Autodesk Inventor part; units mm, degrees
(part 2 of 3)
  line L756 (23.8125, 171.1325) -> (24.4475, 171.1325)
  line L757 (24.4475, 171.1325) -> (24.4475, 171.7675)
  line L758 (23.8125, 171.7675) -> (23.8125, 171.1325)
  line L759 (24.4475, 171.7675) -> (23.8125, 171.7675)
  line L760 (24.4475, 171.7675) -> (23.8125, 171.1325) construction
  line L761 (23.8125, 171.7675) -> (24.4475, 171.1325) construction
  line L762 (26.3525, 171.1325) -> (26.9875, 171.1325)
  line L763 (26.9875, 171.1325) -> (26.9875, 171.7675)
  line L764 (26.3525, 171.7675) -> (26.3525, 171.1325)
  line L765 (26.9875, 171.7675) -> (26.3525, 171.7675)
  line L766 (26.9875, 171.7675) -> (26.3525, 171.1325) construction
  line L767 (26.3525, 171.7675) -> (26.9875, 171.1325) construction
  line L768 (28.8925, 171.1325) -> (29.5275, 171.1325)
  line L769 (29.5275, 171.1325) -> (29.5275, 171.7675)
  line L770 (28.8925, 171.7675) -> (28.8925, 171.1325)
  line L771 (29.5275, 171.7675) -> (28.8925, 171.7675)
  line L772 (29.5275, 171.7675) -> (28.8925, 171.1325) construction
  line L773 (28.8925, 171.7675) -> (29.5275, 171.1325) construction
  line L774 (31.4325, 171.1325) -> (32.0675, 171.1325)
  line L775 (32.0675, 171.1325) -> (32.0675, 171.7675)
  line L776 (31.4325, 171.7675) -> (31.4325, 171.1325)
  line L777 (32.0675, 171.7675) -> (31.4325, 171.7675)
  line L778 (32.0675, 171.7675) -> (31.4325, 171.1325) construction
  line L779 (31.4325, 171.7675) -> (32.0675, 171.1325) construction
  line L780 (33.9725, 171.1325) -> (34.6075, 171.1325)
  line L781 (34.6075, 171.1325) -> (34.6075, 171.7675)
  line L782 (33.9725, 171.7675) -> (33.9725, 171.1325)
  line L783 (34.6075, 171.7675) -> (33.9725, 171.7675)
  line L784 (34.6075, 171.7675) -> (33.9725, 171.1325) construction
  line L785 (33.9725, 171.7675) -> (34.6075, 171.1325) construction
  line L786 (36.5125, 171.1325) -> (37.1475, 171.1325)
  line L787 (37.1475, 171.1325) -> (37.1475, 171.7675)
  line L788 (36.5125, 171.7675) -> (36.5125, 171.1325)
  line L789 (37.1475, 171.7675) -> (36.5125, 171.7675)
  line L790 (37.1475, 171.7675) -> (36.5125, 171.1325) construction
  line L791 (36.5125, 171.7675) -> (37.1475, 171.1325) construction
  line L792 (39.0525, 171.1325) -> (39.6875, 171.1325)
  line L793 (39.6875, 171.1325) -> (39.6875, 171.7675)
  line L794 (39.0525, 171.7675) -> (39.0525, 171.1325)
  line L795 (39.6875, 171.7675) -> (39.0525, 171.7675)
  line L796 (39.6875, 171.7675) -> (39.0525, 171.1325) construction
  line L797 (39.0525, 171.7675) -> (39.6875, 171.1325) construction
  line L798 (169.2275, 37.1475) -> (168.5925, 37.1475)
  line L799 (168.5925, 36.5125) -> (169.2275, 36.5125)
  line L800 (169.2275, 36.5125) -> (169.2275, 37.1475)
  line L801 (169.2275, 37.1475) -> (168.5925, 36.5125) construction
  line L802 (168.5925, 37.1475) -> (169.2275, 36.5125) construction
  line L803 (168.5925, 37.1475) -> (168.5925, 36.5125)
  line L804 (169.2275, 34.6075) -> (168.5925, 34.6075)
  line L805 (168.5925, 33.9725) -> (169.2275, 33.9725)
  line L806 (169.2275, 33.9725) -> (169.2275, 34.6075)
  line L807 (169.2275, 34.6075) -> (168.5925, 33.9725) construction
  line L808 (168.5925, 34.6075) -> (169.2275, 33.9725) construction
  line L809 (168.5925, 34.6075) -> (168.5925, 33.9725)
  line L810 (169.2275, 32.0675) -> (168.5925, 32.0675)
  line L811 (168.5925, 31.4325) -> (169.2275, 31.4325)
  line L812 (169.2275, 31.4325) -> (169.2275, 32.0675)
  line L813 (169.2275, 32.0675) -> (168.5925, 31.4325) construction
  line L814 (168.5925, 32.0675) -> (169.2275, 31.4325) construction
  line L815 (168.5925, 32.0675) -> (168.5925, 31.4325)
  line L816 (169.2275, 29.5275) -> (168.5925, 29.5275)
  line L817 (168.5925, 28.8925) -> (169.2275, 28.8925)
  line L818 (169.2275, 28.8925) -> (169.2275, 29.5275)
  line L819 (169.2275, 29.5275) -> (168.5925, 28.8925) construction
  line L820 (168.5925, 29.5275) -> (169.2275, 28.8925) construction
  line L821 (168.5925, 29.5275) -> (168.5925, 28.8925)
  line L822 (169.2275, 26.9875) -> (168.5925, 26.9875)
  line L823 (168.5925, 26.3525) -> (169.2275, 26.3525)
  line L824 (169.2275, 26.3525) -> (169.2275, 26.9875)
  line L825 (169.2275, 26.9875) -> (168.5925, 26.3525) construction
  line L826 (168.5925, 26.9875) -> (169.2275, 26.3525) construction
  line L827 (168.5925, 26.9875) -> (168.5925, 26.3525)
  line L828 (169.2275, 24.4475) -> (168.5925, 24.4475)
  line L829 (168.5925, 23.8125) -> (169.2275, 23.8125)
  line L830 (169.2275, 23.8125) -> (169.2275, 24.4475)
  line L831 (169.2275, 24.4475) -> (168.5925, 23.8125) construction
  line L832 (168.5925, 24.4475) -> (169.2275, 23.8125) construction
  line L833 (168.5925, 24.4475) -> (168.5925, 23.8125)
  line L834 (169.2275, 21.9075) -> (168.5925, 21.9075)
  line L835 (168.5925, 21.2725) -> (169.2275, 21.2725)
  line L836 (169.2275, 21.2725) -> (169.2275, 21.9075)
  line L837 (169.2275, 21.9075) -> (168.5925, 21.2725) construction
  line L838 (168.5925, 21.9075) -> (169.2275, 21.2725) construction
  line L839 (168.5925, 21.9075) -> (168.5925, 21.2725)
  line L840 (169.2275, 19.3675) -> (168.5925, 19.3675)
  line L841 (168.5925, 18.7325) -> (169.2275, 18.7325)
  line L842 (169.2275, 18.7325) -> (169.2275, 19.3675)
  line L843 (169.2275, 19.3675) -> (168.5925, 18.7325) construction
  line L844 (168.5925, 19.3675) -> (169.2275, 18.7325) construction
  line L845 (168.5925, 19.3675) -> (168.5925, 18.7325)
  line L846 (169.2275, 16.8275) -> (168.5925, 16.8275)
  line L847 (168.5925, 16.1925) -> (169.2275, 16.1925)
  line L848 (169.2275, 16.1925) -> (169.2275, 16.8275)
  line L849 (169.2275, 16.8275) -> (168.5925, 16.1925) construction
  line L850 (168.5925, 16.8275) -> (169.2275, 16.1925) construction
  line L851 (168.5925, 16.8275) -> (168.5925, 16.1925)
  line L852 (169.2275, 14.2875) -> (168.5925, 14.2875)
  line L853 (168.5925, 13.6525) -> (169.2275, 13.6525)
  line L854 (169.2275, 13.6525) -> (169.2275, 14.2875)
  line L855 (169.2275, 14.2875) -> (168.5925, 13.6525) construction
  line L856 (168.5925, 14.2875) -> (169.2275, 13.6525) construction
  line L857 (168.5925, 14.2875) -> (168.5925, 13.6525)
  line L858 (169.2275, 11.7475) -> (168.5925, 11.7475)
  line L859 (168.5925, 11.1125) -> (169.2275, 11.1125)
  line L860 (169.2275, 11.1125) -> (169.2275, 11.7475)
  line L861 (169.2275, 11.7475) -> (168.5925, 11.1125) construction
  line L862 (168.5925, 11.7475) -> (169.2275, 11.1125) construction
  line L863 (168.5925, 11.7475) -> (168.5925, 11.1125)
  line L864 (169.2275, 9.2075) -> (168.5925, 9.2075)
  line L865 (168.5925, 8.5725) -> (169.2275, 8.5725)
  line L866 (169.2275, 8.5725) -> (169.2275, 9.2075)
  line L867 (169.2275, 9.2075) -> (168.5925, 8.5725) construction
  line L868 (168.5925, 9.2075) -> (169.2275, 8.5725) construction
  line L869 (168.5925, 9.2075) -> (168.5925, 8.5725)
  line L870 (169.2275, 6.6675) -> (168.5925, 6.6675)
  line L871 (168.5925, 6.0325) -> (169.2275, 6.0325)
  line L872 (169.2275, 6.0325) -> (169.2275, 6.6675)
  line L873 (169.2275, 6.6675) -> (168.5925, 6.0325) construction
  line L874 (168.5925, 6.6675) -> (169.2275, 6.0325) construction
  line L875 (168.5925, 6.6675) -> (168.5925, 6.0325)
  line L876 (169.2275, 4.1275) -> (168.5925, 4.1275)
  line L877 (168.5925, 3.4925) -> (169.2275, 3.4925)
  line L878 (169.2275, 3.4925) -> (169.2275, 4.1275)
  line L879 (169.2275, 4.1275) -> (168.5925, 3.4925) construction
  line L880 (168.5925, 4.1275) -> (169.2275, 3.4925) construction
  line L881 (168.5925, 4.1275) -> (168.5925, 3.4925)
  line L882 (169.2275, 1.5875) -> (168.5925, 1.5875)
  line L883 (168.5925, 0.9525) -> (169.2275, 0.9525)
  line L884 (169.2275, 0.9525) -> (169.2275, 1.5875)
  line L885 (169.2275, 1.5875) -> (168.5925, 0.9525) construction
  line L886 (168.5925, 1.5875) -> (169.2275, 0.9525) construction
  line L887 (168.5925, 1.5875) -> (168.5925, 0.9525)
  line L888 (169.2275, -0.9525) -> (168.5925, -0.9525)
  line L889 (168.5925, -1.5875) -> (169.2275, -1.5875)
  line L890 (169.2275, -1.5875) -> (169.2275, -0.9525)
  line L891 (169.2275, -0.9525) -> (168.5925, -1.5875) construction
  line L892 (168.5925, -0.9525) -> (169.2275, -1.5875) construction
  line L893 (168.5925, -0.9525) -> (168.5925, -1.5875)
  line L894 (169.2275, -3.4925) -> (168.5925, -3.4925)
  line L895 (168.5925, -4.1275) -> (169.2275, -4.1275)
  line L896 (169.2275, -4.1275) -> (169.2275, -3.4925)
  line L897 (169.2275, -3.4925) -> (168.5925, -4.1275) construction
  line L898 (168.5925, -3.4925) -> (169.2275, -4.1275) construction
  line L899 (168.5925, -3.4925) -> (168.5925, -4.1275)
  line L900 (169.2275, -6.0325) -> (168.5925, -6.0325)
  line L901 (168.5925, -6.6675) -> (169.2275, -6.6675)
  line L902 (169.2275, -6.6675) -> (169.2275, -6.0325)
  line L903 (169.2275, -6.0325) -> (168.5925, -6.6675) construction
  line L904 (168.5925, -6.0325) -> (169.2275, -6.6675) construction
  line L905 (168.5925, -6.0325) -> (168.5925, -6.6675)
  line L906 (169.2275, -8.5725) -> (168.5925, -8.5725)
  line L907 (168.5925, -9.2075) -> (169.2275, -9.2075)
  line L908 (169.2275, -9.2075) -> (169.2275, -8.5725)
  line L909 (169.2275, -8.5725) -> (168.5925, -9.2075) construction
  line L910 (168.5925, -8.5725) -> (169.2275, -9.2075) construction
  line L911 (168.5925, -8.5725) -> (168.5925, -9.2075)
  line L912 (169.2275, -11.1125) -> (168.5925, -11.1125)
  line L913 (168.5925, -11.7475) -> (169.2275, -11.7475)
  line L914 (169.2275, -11.7475) -> (169.2275, -11.1125)
  line L915 (169.2275, -11.1125) -> (168.5925, -11.7475) construction
  line L916 (168.5925, -11.1125) -> (169.2275, -11.7475) construction
  line L917 (168.5925, -11.1125) -> (168.5925, -11.7475)
  line L918 (169.2275, -13.6525) -> (168.5925, -13.6525)
  line L919 (168.5925, -14.2875) -> (169.2275, -14.2875)
  line L920 (169.2275, -14.2875) -> (169.2275, -13.6525)
  line L921 (169.2275, -13.6525) -> (168.5925, -14.2875) construction
  line L922 (168.5925, -13.6525) -> (169.2275, -14.2875) construction
  line L923 (168.5925, -13.6525) -> (168.5925, -14.2875)
  line L924 (169.2275, -16.1925) -> (168.5925, -16.1925)
  line L925 (168.5925, -16.8275) -> (169.2275, -16.8275)
  line L926 (169.2275, -16.8275) -> (169.2275, -16.1925)
  line L927 (169.2275, -16.1925) -> (168.5925, -16.8275) construction
  line L928 (168.5925, -16.1925) -> (169.2275, -16.8275) construction
  line L929 (168.5925, -16.1925) -> (168.5925, -16.8275)
  line L930 (169.2275, -18.7325) -> (168.5925, -18.7325)
  line L931 (168.5925, -19.3675) -> (169.2275, -19.3675)
  line L932 (169.2275, -19.3675) -> (169.2275, -18.7325)
  line L933 (169.2275, -18.7325) -> (168.5925, -19.3675) construction
  line L934 (168.5925, -18.7325) -> (169.2275, -19.3675) construction
  line L935 (168.5925, -18.7325) -> (168.5925, -19.3675)
  line L936 (169.2275, -21.2725) -> (168.5925, -21.2725)
  line L937 (168.5925, -21.9075) -> (169.2275, -21.9075)
  line L938 (169.2275, -21.9075) -> (169.2275, -21.2725)
  line L939 (169.2275, -21.2725) -> (168.5925, -21.9075) construction
  line L940 (168.5925, -21.2725) -> (169.2275, -21.9075) construction
  line L941 (168.5925, -21.2725) -> (168.5925, -21.9075)
  line L942 (169.2275, -23.8125) -> (168.5925, -23.8125)
  line L943 (168.5925, -24.4475) -> (169.2275, -24.4475)
  line L944 (169.2275, -24.4475) -> (169.2275, -23.8125)
  line L945 (169.2275, -23.8125) -> (168.5925, -24.4475) construction
  line L946 (168.5925, -23.8125) -> (169.2275, -24.4475) construction
  line L947 (168.5925, -23.8125) -> (168.5925, -24.4475)
  line L948 (169.2275, -26.3525) -> (168.5925, -26.3525)
  line L949 (168.5925, -26.9875) -> (169.2275, -26.9875)
  line L950 (169.2275, -26.9875) -> (169.2275, -26.3525)
  line L951 (169.2275, -26.3525) -> (168.5925, -26.9875) construction
  line L952 (168.5925, -26.3525) -> (169.2275, -26.9875) construction
  line L953 (168.5925, -26.3525) -> (168.5925, -26.9875)
  line L954 (169.2275, -28.8925) -> (168.5925, -28.8925)
  line L955 (168.5925, -29.5275) -> (169.2275, -29.5275)
  line L956 (169.2275, -29.5275) -> (169.2275, -28.8925)
  line L957 (169.2275, -28.8925) -> (168.5925, -29.5275) construction
  line L958 (168.5925, -28.8925) -> (169.2275, -29.5275) construction
  line L959 (168.5925, -28.8925) -> (168.5925, -29.5275)
  line L960 (169.2275, -31.4325) -> (168.5925, -31.4325)
  line L961 (168.5925, -32.0675) -> (169.2275, -32.0675)
  line L962 (169.2275, -32.0675) -> (169.2275, -31.4325)
  line L963 (169.2275, -31.4325) -> (168.5925, -32.0675) construction
  line L964 (168.5925, -31.4325) -> (169.2275, -32.0675) construction
  line L965 (168.5925, -31.4325) -> (168.5925, -32.0675)
  line L966 (169.2275, -33.9725) -> (168.5925, -33.9725)
  line L967 (168.5925, -34.6075) -> (169.2275, -34.6075)
  line L968 (169.2275, -34.6075) -> (169.2275, -33.9725)
  line L969 (169.2275, -33.9725) -> (168.5925, -34.6075) construction
  line L970 (168.5925, -33.9725) -> (169.2275, -34.6075) construction
  line L971 (168.5925, -33.9725) -> (168.5925, -34.6075)
  line L972 (169.2275, -36.5125) -> (168.5925, -36.5125)
  line L973 (168.5925, -37.1475) -> (169.2275, -37.1475)
  line L974 (169.2275, -37.1475) -> (169.2275, -36.5125)
  line L975 (169.2275, -36.5125) -> (168.5925, -37.1475) construction
  line L976 (168.5925, -36.5125) -> (169.2275, -37.1475) construction
  line L977 (168.5925, -36.5125) -> (168.5925, -37.1475)
  line L978 (169.2275, -39.0525) -> (168.5925, -39.0525)
  line L979 (168.5925, -39.6875) -> (169.2275, -39.6875)
  line L980 (169.2275, -39.6875) -> (169.2275, -39.0525)
  line L981 (169.2275, -39.0525) -> (168.5925, -39.6875) construction
  line L982 (168.5925, -39.0525) -> (169.2275, -39.6875) construction
  line L983 (168.5925, -39.0525) -> (168.5925, -39.6875)
  line L984 (171.7675, 39.6875) -> (171.1325, 39.6875)
  line L985 (171.1325, 39.0525) -> (171.7675, 39.0525)
  line L986 (171.7675, 39.0525) -> (171.7675, 39.6875)
  line L987 (171.7675, 39.6875) -> (171.1325, 39.0525) construction
  line L988 (171.1325, 39.6875) -> (171.7675, 39.0525) construction
  line L989 (171.1325, 39.6875) -> (171.1325, 39.0525)
  line L990 (171.7675, 37.1475) -> (171.1325, 37.1475)
  line L991 (171.1325, 36.5125) -> (171.7675, 36.5125)
  line L992 (171.7675, 36.5125) -> (171.7675, 37.1475)
  line L993 (171.7675, 37.1475) -> (171.1325, 36.5125) construction
  line L994 (171.1325, 37.1475) -> (171.7675, 36.5125) construction
  line L995 (171.1325, 37.1475) -> (171.1325, 36.5125)
  line L996 (171.7675, 34.6075) -> (171.1325, 34.6075)
  line L997 (171.1325, 33.9725) -> (171.7675, 33.9725)
  line L998 (171.7675, 33.9725) -> (171.7675, 34.6075)
  line L999 (171.7675, 34.6075) -> (171.1325, 33.9725) construction
  line L1000 (171.1325, 34.6075) -> (171.7675, 33.9725) construction
  line L1001 (171.1325, 34.6075) -> (171.1325, 33.9725)
  line L1002 (171.7675, 32.0675) -> (171.1325, 32.0675)
  line L1003 (171.1325, 31.4325) -> (171.7675, 31.4325)
  line L1004 (171.7675, 31.4325) -> (171.7675, 32.0675)
  line L1005 (171.7675, 32.0675) -> (171.1325, 31.4325) construction
  line L1006 (171.1325, 32.0675) -> (171.7675, 31.4325) construction
  line L1007 (171.1325, 32.0675) -> (171.1325, 31.4325)
  line L1008 (171.7675, 29.5275) -> (171.1325, 29.5275)
  line L1009 (171.1325, 28.8925) -> (171.7675, 28.8925)
  line L1010 (171.7675, 28.8925) -> (171.7675, 29.5275)
  line L1011 (171.7675, 29.5275) -> (171.1325, 28.8925) construction
  line L1012 (171.1325, 29.5275) -> (171.7675, 28.8925) construction
  line L1013 (171.1325, 29.5275) -> (171.1325, 28.8925)
  line L1014 (171.7675, 26.9875) -> (171.1325, 26.9875)
  line L1015 (171.1325, 26.3525) -> (171.7675, 26.3525)
  line L1016 (171.7675, 26.3525) -> (171.7675, 26.9875)
  line L1017 (171.7675, 26.9875) -> (171.1325, 26.3525) construction
  line L1018 (171.1325, 26.9875) -> (171.7675, 26.3525) construction
  line L1019 (171.1325, 26.9875) -> (171.1325, 26.3525)
  line L1020 (171.7675, 24.4475) -> (171.1325, 24.4475)
  line L1021 (171.1325, 23.8125) -> (171.7675, 23.8125)
  line L1022 (171.7675, 23.8125) -> (171.7675, 24.4475)
  line L1023 (171.7675, 24.4475) -> (171.1325, 23.8125) construction
  line L1024 (171.1325, 24.4475) -> (171.7675, 23.8125) construction
  line L1025 (171.1325, 24.4475) -> (171.1325, 23.8125)
  line L1026 (171.7675, 21.9075) -> (171.1325, 21.9075)
  line L1027 (171.1325, 21.2725) -> (171.7675, 21.2725)
  line L1028 (171.7675, 21.2725) -> (171.7675, 21.9075)
  line L1029 (171.7675, 21.9075) -> (171.1325, 21.2725) construction
  line L1030 (171.1325, 21.9075) -> (171.7675, 21.2725) construction
  line L1031 (171.1325, 21.9075) -> (171.1325, 21.2725)
  line L1032 (171.7675, 19.3675) -> (171.1325, 19.3675)
  line L1033 (171.1325, 18.7325) -> (171.7675, 18.7325)
  line L1034 (171.7675, 18.7325) -> (171.7675, 19.3675)
  line L1035 (171.7675, 19.3675) -> (171.1325, 18.7325) construction
  line L1036 (171.1325, 19.3675) -> (171.7675, 18.7325) construction
  line L1037 (171.1325, 19.3675) -> (171.1325, 18.7325)
  line L1038 (171.7675, 16.8275) -> (171.1325, 16.8275)
  line L1039 (171.1325, 16.1925) -> (171.7675, 16.1925)
  line L1040 (171.7675, 16.1925) -> (171.7675, 16.8275)
  line L1041 (171.7675, 16.8275) -> (171.1325, 16.1925) construction
  line L1042 (171.1325, 16.8275) -> (171.7675, 16.1925) construction
  line L1043 (171.1325, 16.8275) -> (171.1325, 16.1925)
  line L1044 (171.7675, 14.2875) -> (171.1325, 14.2875)
  line L1045 (171.1325, 13.6525) -> (171.7675, 13.6525)
  line L1046 (171.7675, 13.6525) -> (171.7675, 14.2875)
  line L1047 (171.7675, 14.2875) -> (171.1325, 13.6525) construction
  line L1048 (171.1325, 14.2875) -> (171.7675, 13.6525) construction
  line L1049 (171.1325, 14.2875) -> (171.1325, 13.6525)
  line L1050 (171.7675, 11.7475) -> (171.1325, 11.7475)
  line L1051 (171.1325, 11.1125) -> (171.7675, 11.1125)
  line L1052 (171.7675, 11.1125) -> (171.7675, 11.7475)
  line L1053 (171.7675, 11.7475) -> (171.1325, 11.1125) construction
  line L1054 (171.1325, 11.7475) -> (171.7675, 11.1125) construction
  line L1055 (171.1325, 11.7475) -> (171.1325, 11.1125)
  line L1056 (171.7675, 9.2075) -> (171.1325, 9.2075)
  line L1057 (171.1325, 8.5725) -> (171.7675, 8.5725)
  line L1058 (171.7675, 8.5725) -> (171.7675, 9.2075)
  line L1059 (171.7675, 9.2075) -> (171.1325, 8.5725) construction
  line L1060 (171.1325, 9.2075) -> (171.7675, 8.5725) construction
  line L1061 (171.1325, 9.2075) -> (171.1325, 8.5725)
  line L1062 (171.7675, 6.6675) -> (171.1325, 6.6675)
  line L1063 (171.1325, 6.0325) -> (171.7675, 6.0325)
  line L1064 (171.7675, 6.0325) -> (171.7675, 6.6675)
  line L1065 (171.7675, 6.6675) -> (171.1325, 6.0325) construction
  line L1066 (171.1325, 6.6675) -> (171.7675, 6.0325) construction
  line L1067 (171.1325, 6.6675) -> (171.1325, 6.0325)
  line L1068 (171.7675, 4.1275) -> (171.1325, 4.1275)
  line L1069 (171.1325, 3.4925) -> (171.7675, 3.4925)
  line L1070 (171.7675, 3.4925) -> (171.7675, 4.1275)
  line L1071 (171.7675, 4.1275) -> (171.1325, 3.4925) construction
  line L1072 (171.1325, 4.1275) -> (171.7675, 3.4925) construction
  line L1073 (171.1325, 4.1275) -> (171.1325, 3.4925)
  line L1074 (171.7675, 1.5875) -> (171.1325, 1.5875)
  line L1075 (171.1325, 0.9525) -> (171.7675, 0.9525)
  line L1076 (171.7675, 0.9525) -> (171.7675, 1.5875)
  line L1077 (171.7675, 1.5875) -> (171.1325, 0.9525) construction
  line L1078 (171.1325, 1.5875) -> (171.7675, 0.9525) construction
  line L1079 (171.1325, 1.5875) -> (171.1325, 0.9525)
  line L1080 (171.7675, -0.9525) -> (171.1325, -0.9525)
  line L1081 (171.1325, -1.5875) -> (171.7675, -1.5875)
  line L1082 (171.7675, -1.5875) -> (171.7675, -0.9525)
  line L1083 (171.7675, -0.9525) -> (171.1325, -1.5875) construction
  line L1084 (171.1325, -0.9525) -> (171.7675, -1.5875) construction
  line L1085 (171.1325, -0.9525) -> (171.1325, -1.5875)
  line L1086 (171.7675, -3.4925) -> (171.1325, -3.4925)
  line L1087 (171.1325, -4.1275) -> (171.7675, -4.1275)
  line L1088 (171.7675, -4.1275) -> (171.7675, -3.4925)
  line L1089 (171.7675, -3.4925) -> (171.1325, -4.1275) construction
  line L1090 (171.1325, -3.4925) -> (171.7675, -4.1275) construction
  line L1091 (171.1325, -3.4925) -> (171.1325, -4.1275)
  line L1092 (171.7675, -6.0325) -> (171.1325, -6.0325)
  line L1093 (171.1325, -6.6675) -> (171.7675, -6.6675)
  line L1094 (171.7675, -6.6675) -> (171.7675, -6.0325)
  line L1095 (171.7675, -6.0325) -> (171.1325, -6.6675) construction
  line L1096 (171.1325, -6.0325) -> (171.7675, -6.6675) construction
  line L1097 (171.1325, -6.0325) -> (171.1325, -6.6675)
  line L1098 (171.7675, -8.5725) -> (171.1325, -8.5725)
  line L1099 (171.1325, -9.2075) -> (171.7675, -9.2075)
  line L1100 (171.7675, -9.2075) -> (171.7675, -8.5725)
  line L1101 (171.7675, -8.5725) -> (171.1325, -9.2075) construction
  line L1102 (171.1325, -8.5725) -> (171.7675, -9.2075) construction
  line L1103 (171.1325, -8.5725) -> (171.1325, -9.2075)
  line L1104 (171.7675, -11.1125) -> (171.1325, -11.1125)
  line L1105 (171.1325, -11.7475) -> (171.7675, -11.7475)
  line L1106 (171.7675, -11.7475) -> (171.7675, -11.1125)
  line L1107 (171.7675, -11.1125) -> (171.1325, -11.7475) construction
  line L1108 (171.1325, -11.1125) -> (171.7675, -11.7475) construction
  line L1109 (171.1325, -11.1125) -> (171.1325, -11.7475)
  line L1110 (171.7675, -13.6525) -> (171.1325, -13.6525)
  line L1111 (171.1325, -14.2875) -> (171.7675, -14.2875)
  line L1112 (171.7675, -14.2875) -> (171.7675, -13.6525)
  line L1113 (171.7675, -13.6525) -> (171.1325, -14.2875) construction
  line L1114 (171.1325, -13.6525) -> (171.7675, -14.2875) construction
  line L1115 (171.1325, -13.6525) -> (171.1325, -14.2875)
  line L1116 (171.7675, -16.1925) -> (171.1325, -16.1925)
  line L1117 (171.1325, -16.8275) -> (171.7675, -16.8275)
  line L1118 (171.7675, -16.8275) -> (171.7675, -16.1925)
  line L1119 (171.7675, -16.1925) -> (171.1325, -16.8275) construction
  line L1120 (171.1325, -16.1925) -> (171.7675, -16.8275) construction
  line L1121 (171.1325, -16.1925) -> (171.1325, -16.8275)
  line L1122 (171.7675, -18.7325) -> (171.1325, -18.7325)
  line L1123 (171.1325, -19.3675) -> (171.7675, -19.3675)
  line L1124 (171.7675, -19.3675) -> (171.7675, -18.7325)
  line L1125 (171.7675, -18.7325) -> (171.1325, -19.3675) construction
  line L1126 (171.1325, -18.7325) -> (171.7675, -19.3675) construction
  line L1127 (171.1325, -18.7325) -> (171.1325, -19.3675)
  line L1128 (171.7675, -21.2725) -> (171.1325, -21.2725)
  line L1129 (171.1325, -21.9075) -> (171.7675, -21.9075)
  line L1130 (171.7675, -21.9075) -> (171.7675, -21.2725)
  line L1131 (171.7675, -21.2725) -> (171.1325, -21.9075) construction
  line L1132 (171.1325, -21.2725) -> (171.7675, -21.9075) construction
  line L1133 (171.1325, -21.2725) -> (171.1325, -21.9075)
  line L1134 (171.7675, -23.8125) -> (171.1325, -23.8125)
  line L1135 (171.1325, -24.4475) -> (171.7675, -24.4475)
  line L1136 (171.7675, -24.4475) -> (171.7675, -23.8125)
  line L1137 (171.7675, -23.8125) -> (171.1325, -24.4475) construction
  line L1138 (171.1325, -23.8125) -> (171.7675, -24.4475) construction
  line L1139 (171.1325, -23.8125) -> (171.1325, -24.4475)
  line L1140 (171.7675, -26.3525) -> (171.1325, -26.3525)
  line L1141 (171.1325, -26.9875) -> (171.7675, -26.9875)
  line L1142 (171.7675, -26.9875) -> (171.7675, -26.3525)
  line L1143 (171.7675, -26.3525) -> (171.1325, -26.9875) construction
  line L1144 (171.1325, -26.3525) -> (171.7675, -26.9875) construction
  line L1145 (171.1325, -26.3525) -> (171.1325, -26.9875)
  line L1146 (171.7675, -28.8925) -> (171.1325, -28.8925)
  line L1147 (171.1325, -29.5275) -> (171.7675, -29.5275)
  line L1148 (171.7675, -29.5275) -> (171.7675, -28.8925)
  line L1149 (171.7675, -28.8925) -> (171.1325, -29.5275) construction
  line L1150 (171.1325, -28.8925) -> (171.7675, -29.5275) construction
  line L1151 (171.1325, -28.8925) -> (171.1325, -29.5275)
  line L1152 (171.7675, -31.4325) -> (171.1325, -31.4325)
  line L1153 (171.1325, -32.0675) -> (171.7675, -32.0675)
  line L1154 (171.7675, -32.0675) -> (171.7675, -31.4325)
  line L1155 (171.7675, -31.4325) -> (171.1325, -32.0675) construction
  line L1156 (171.1325, -31.4325) -> (171.7675, -32.0675) construction
  line L1157 (171.1325, -31.4325) -> (171.1325, -32.0675)
  line L1158 (171.7675, -33.9725) -> (171.1325, -33.9725)
  line L1159 (171.1325, -34.6075) -> (171.7675, -34.6075)
  line L1160 (171.7675, -34.6075) -> (171.7675, -33.9725)
  line L1161 (171.7675, -33.9725) -> (171.1325, -34.6075) construction
  line L1162 (171.1325, -33.9725) -> (171.7675, -34.6075) construction
  line L1163 (171.1325, -33.9725) -> (171.1325, -34.6075)
  line L1164 (171.7675, -36.5125) -> (171.1325, -36.5125)
  line L1165 (171.1325, -37.1475) -> (171.7675, -37.1475)
  line L1166 (171.7675, -37.1475) -> (171.7675, -36.5125)
  line L1167 (171.7675, -36.5125) -> (171.1325, -37.1475) construction
  line L1168 (171.1325, -36.5125) -> (171.7675, -37.1475) construction
  line L1169 (171.1325, -36.5125) -> (171.1325, -37.1475)
  line L1170 (171.7675, -39.0525) -> (171.1325, -39.0525)
  line L1171 (171.1325, -39.6875) -> (171.7675, -39.6875)
  line L1172 (171.7675, -39.6875) -> (171.7675, -39.0525)
  line L1173 (171.7675, -39.0525) -> (171.1325, -39.6875) construction
  line L1174 (171.1325, -39.0525) -> (171.7675, -39.6875) construction
  line L1175 (171.1325, -39.0525) -> (171.1325, -39.6875)
  line L1176 (-172.72, -40.64) -> (-167.64, -40.64)
  line L1177 (-167.64, -40.64) -> (-167.64, 40.64)
  line L1178 (-167.64, 40.64) -> (-172.72, 40.64)
  line L1179 (-172.72, 40.64) -> (-172.72, -40.64)
  line L1180 (-169.2275, 39.6875) -> (-168.5925, 39.6875)
  line L1181 (-168.5925, 39.6875) -> (-168.5925, 39.0525)
  line L1182 (-168.5925, 39.0525) -> (-169.2275, 39.0525)
  line L1183 (-169.2275, 39.0525) -> (-169.2275, 39.6875)
  line L1184 (-168.5925, 36.5125) -> (-169.2275, 36.5125)
  line L1185 (-169.2275, 36.5125) -> (-169.2275, 37.1475)
  line L1186 (-169.2275, 37.1475) -> (-168.5925, 37.1475)
  line L1187 (-168.5925, 37.1475) -> (-168.5925, 36.5125)
  line L1188 (-168.5925, 33.9725) -> (-169.2275, 33.9725)
  line L1189 (-169.2275, 33.9725) -> (-169.2275, 34.6075)
  line L1190 (-169.2275, 34.6075) -> (-168.5925, 34.6075)
  line L1191 (-168.5925, 34.6075) -> (-168.5925, 33.9725)
  line L1192 (-168.5925, 31.4325) -> (-169.2275, 31.4325)
  line L1193 (-169.2275, 31.4325) -> (-169.2275, 32.0675)
  line L1194 (-169.2275, 32.0675) -> (-168.5925, 32.0675)
  line L1195 (-168.5925, 32.0675) -> (-168.5925, 31.4325)
  line L1196 (-168.5925, 28.8925) -> (-169.2275, 28.8925)
  line L1197 (-169.2275, 28.8925) -> (-169.2275, 29.5275)
  line L1198 (-169.2275, 29.5275) -> (-168.5925, 29.5275)
  line L1199 (-168.5925, 29.5275) -> (-168.5925, 28.8925)
  line L1200 (-168.5925, 26.3525) -> (-169.2275, 26.3525)
  line L1201 (-169.2275, 26.3525) -> (-169.2275, 26.9875)
  line L1202 (-169.2275, 26.9875) -> (-168.5925, 26.9875)
  line L1203 (-168.5925, 26.9875) -> (-168.5925, 26.3525)
  line L1204 (-168.5925, 23.8125) -> (-169.2275, 23.8125)
  line L1205 (-169.2275, 23.8125) -> (-169.2275, 24.4475)
  line L1206 (-169.2275, 24.4475) -> (-168.5925, 24.4475)
  line L1207 (-168.5925, 24.4475) -> (-168.5925, 23.8125)
  line L1208 (-168.5925, 21.2725) -> (-169.2275, 21.2725)
  line L1209 (-169.2275, 21.2725) -> (-169.2275, 21.9075)
  line L1210 (-169.2275, 21.9075) -> (-168.5925, 21.9075)
  line L1211 (-168.5925, 21.9075) -> (-168.5925, 21.2725)
  line L1212 (-168.5925, 18.7325) -> (-169.2275, 18.7325)
  line L1213 (-169.2275, 18.7325) -> (-169.2275, 19.3675)
  line L1214 (-169.2275, 19.3675) -> (-168.5925, 19.3675)
  line L1215 (-168.5925, 19.3675) -> (-168.5925, 18.7325)
  line L1216 (-168.5925, 16.1925) -> (-169.2275, 16.1925)
  line L1217 (-169.2275, 16.1925) -> (-169.2275, 16.8275)
  line L1218 (-169.2275, 16.8275) -> (-168.5925, 16.8275)
  line L1219 (-168.5925, 16.8275) -> (-168.5925, 16.1925)
  line L1220 (-168.5925, 13.6525) -> (-169.2275, 13.6525)
  line L1221 (-169.2275, 13.6525) -> (-169.2275, 14.2875)
  line L1222 (-169.2275, 14.2875) -> (-168.5925, 14.2875)
  line L1223 (-168.5925, 14.2875) -> (-168.5925, 13.6525)
  line L1224 (-168.5925, 11.1125) -> (-169.2275, 11.1125)
  line L1225 (-169.2275, 11.1125) -> (-169.2275, 11.7475)
  line L1226 (-169.2275, 11.7475) -> (-168.5925, 11.7475)
  line L1227 (-168.5925, 11.7475) -> (-168.5925, 11.1125)
  line L1228 (-168.5925, 8.5725) -> (-169.2275, 8.5725)
  line L1229 (-169.2275, 8.5725) -> (-169.2275, 9.2075)
  line L1230 (-169.2275, 9.2075) -> (-168.5925, 9.2075)
  line L1231 (-168.5925, 9.2075) -> (-168.5925, 8.5725)
  line L1232 (-168.5925, 6.0325) -> (-169.2275, 6.0325)
  line L1233 (-169.2275, 6.0325) -> (-169.2275, 6.6675)
  line L1234 (-169.2275, 6.6675) -> (-168.5925, 6.6675)
  line L1235 (-168.5925, 6.6675) -> (-168.5925, 6.0325)
  line L1236 (-168.5925, 3.4925) -> (-169.2275, 3.4925)
  line L1237 (-169.2275, 3.4925) -> (-169.2275, 4.1275)
  line L1238 (-169.2275, 4.1275) -> (-168.5925, 4.1275)
  line L1239 (-168.5925, 4.1275) -> (-168.5925, 3.4925)
  line L1240 (-168.5925, 0.9525) -> (-169.2275, 0.9525)
  line L1241 (-169.2275, 0.9525) -> (-169.2275, 1.5875)
  line L1242 (-169.2275, 1.5875) -> (-168.5925, 1.5875)
  line L1243 (-168.5925, 1.5875) -> (-168.5925, 0.9525)
  line L1244 (-168.5925, -1.5875) -> (-169.2275, -1.5875)
  line L1245 (-169.2275, -1.5875) -> (-169.2275, -0.9525)
  line L1246 (-169.2275, -0.9525) -> (-168.5925, -0.9525)
  line L1247 (-168.5925, -0.9525) -> (-168.5925, -1.5875)
  line L1248 (-168.5925, -4.1275) -> (-169.2275, -4.1275)
  line L1249 (-169.2275, -4.1275) -> (-169.2275, -3.4925)
  line L1250 (-169.2275, -3.4925) -> (-168.5925, -3.4925)
  line L1251 (-168.5925, -3.4925) -> (-168.5925, -4.1275)
  line L1252 (-168.5925, -6.6675) -> (-169.2275, -6.6675)
  line L1253 (-169.2275, -6.6675) -> (-169.2275, -6.0325)
  line L1254 (-169.2275, -6.0325) -> (-168.5925, -6.0325)
  line L1255 (-168.5925, -6.0325) -> (-168.5925, -6.6675)
  line L1256 (-168.5925, -9.2075) -> (-169.2275, -9.2075)
  line L1257 (-169.2275, -9.2075) -> (-169.2275, -8.5725)
  line L1258 (-169.2275, -8.5725) -> (-168.5925, -8.5725)
  line L1259 (-168.5925, -8.5725) -> (-168.5925, -9.2075)
  line L1260 (-168.5925, -11.7475) -> (-169.2275, -11.7475)
  line L1261 (-169.2275, -11.7475) -> (-169.2275, -11.1125)
  line L1262 (-169.2275, -11.1125) -> (-168.5925, -11.1125)
  line L1263 (-168.5925, -11.1125) -> (-168.5925, -11.7475)
  line L1264 (-168.5925, -14.2875) -> (-169.2275, -14.2875)
  line L1265 (-169.2275, -14.2875) -> (-169.2275, -13.6525)
  line L1266 (-169.2275, -13.6525) -> (-168.5925, -13.6525)
  line L1267 (-168.5925, -13.6525) -> (-168.5925, -14.2875)
  line L1268 (-168.5925, -16.8275) -> (-169.2275, -16.8275)
  line L1269 (-169.2275, -16.8275) -> (-169.2275, -16.1925)
  line L1270 (-169.2275, -16.1925) -> (-168.5925, -16.1925)
  line L1271 (-168.5925, -16.1925) -> (-168.5925, -16.8275)
  line L1272 (-168.5925, -19.3675) -> (-169.2275, -19.3675)
  line L1273 (-169.2275, -19.3675) -> (-169.2275, -18.7325)
  line L1274 (-169.2275, -18.7325) -> (-168.5925, -18.7325)
  line L1275 (-168.5925, -18.7325) -> (-168.5925, -19.3675)
  line L1276 (-168.5925, -21.9075) -> (-169.2275, -21.9075)
  line L1277 (-169.2275, -21.9075) -> (-169.2275, -21.2725)
  line L1278 (-169.2275, -21.2725) -> (-168.5925, -21.2725)
  line L1279 (-168.5925, -21.2725) -> (-168.5925, -21.9075)
  line L1280 (-168.5925, -24.4475) -> (-169.2275, -24.4475)
  line L1281 (-169.2275, -24.4475) -> (-169.2275, -23.8125)
  line L1282 (-169.2275, -23.8125) -> (-168.5925, -23.8125)
  line L1283 (-168.5925, -23.8125) -> (-168.5925, -24.4475)
  line L1284 (-168.5925, -26.9875) -> (-169.2275, -26.9875)
  line L1285 (-169.2275, -26.9875) -> (-169.2275, -26.3525)
  line L1286 (-169.2275, -26.3525) -> (-168.5925, -26.3525)
  line L1287 (-168.5925, -26.3525) -> (-168.5925, -26.9875)
  line L1288 (-168.5925, -29.5275) -> (-169.2275, -29.5275)
  line L1289 (-169.2275, -29.5275) -> (-169.2275, -28.8925)
  line L1290 (-169.2275, -28.8925) -> (-168.5925, -28.8925)
  line L1291 (-168.5925, -28.8925) -> (-168.5925, -29.5275)
  line L1292 (-168.5925, -32.0675) -> (-169.2275, -32.0675)
  line L1293 (-169.2275, -32.0675) -> (-169.2275, -31.4325)
  line L1294 (-169.2275, -31.4325) -> (-168.5925, -31.4325)
  line L1295 (-168.5925, -31.4325) -> (-168.5925, -32.0675)
  line L1296 (-168.5925, -34.6075) -> (-169.2275, -34.6075)
  line L1297 (-169.2275, -34.6075) -> (-169.2275, -33.9725)
  line L1298 (-169.2275, -33.9725) -> (-168.5925, -33.9725)
  line L1299 (-168.5925, -33.9725) -> (-168.5925, -34.6075)
  line L1300 (-168.5925, -37.1475) -> (-169.2275, -37.1475)
  line L1301 (-169.2275, -37.1475) -> (-169.2275, -36.5125)
  line L1302 (-169.2275, -36.5125) -> (-168.5925, -36.5125)
  line L1303 (-168.5925, -36.5125) -> (-168.5925, -37.1475)
  line L1304 (-168.5925, -39.6875) -> (-169.2275, -39.6875)
  line L1305 (-169.2275, -39.6875) -> (-169.2275, -39.0525)
  line L1306 (-169.2275, -39.0525) -> (-168.5925, -39.0525)
  line L1307 (-168.5925, -39.0525) -> (-168.5925, -39.6875)
  line L1308 (-171.1325, 39.0525) -> (-171.7675, 39.0525)
  line L1309 (-171.7675, 39.0525) -> (-171.7675, 39.6875)
  line L1310 (-171.7675, 39.6875) -> (-171.1325, 39.6875)
  line L1311 (-171.1325, 39.6875) -> (-171.1325, 39.0525)
  line L1312 (-171.1325, 36.5125) -> (-171.7675, 36.5125)
  line L1313 (-171.7675, 36.5125) -> (-171.7675, 37.1475)
  line L1314 (-171.7675, 37.1475) -> (-171.1325, 37.1475)
  line L1315 (-171.1325, 37.1475) -> (-171.1325, 36.5125)
  line L1316 (-171.1325, 33.9725) -> (-171.7675, 33.9725)
  line L1317 (-171.7675, 33.9725) -> (-171.7675, 34.6075)
  line L1318 (-171.7675, 34.6075) -> (-171.1325, 34.6075)
  line L1319 (-171.1325, 34.6075) -> (-171.1325, 33.9725)
  line L1320 (-171.1325, 31.4325) -> (-171.7675, 31.4325)
  line L1321 (-171.7675, 31.4325) -> (-171.7675, 32.0675)
  line L1322 (-171.7675, 32.0675) -> (-171.1325, 32.0675)
  line L1323 (-171.1325, 32.0675) -> (-171.1325, 31.4325)
  line L1324 (-171.1325, 28.8925) -> (-171.7675, 28.8925)
  line L1325 (-171.7675, 28.8925) -> (-171.7675, 29.5275)
  line L1326 (-171.7675, 29.5275) -> (-171.1325, 29.5275)
  line L1327 (-171.1325, 29.5275) -> (-171.1325, 28.8925)
  line L1328 (-171.1325, 26.3525) -> (-171.7675, 26.3525)
  line L1329 (-171.7675, 26.3525) -> (-171.7675, 26.9875)
  line L1330 (-171.7675, 26.9875) -> (-171.1325, 26.9875)
  line L1331 (-171.1325, 26.9875) -> (-171.1325, 26.3525)
  line L1332 (-171.1325, 23.8125) -> (-171.7675, 23.8125)
  line L1333 (-171.7675, 23.8125) -> (-171.7675, 24.4475)
  line L1334 (-171.7675, 24.4475) -> (-171.1325, 24.4475)
  line L1335 (-171.1325, 24.4475) -> (-171.1325, 23.8125)
  line L1336 (-171.1325, 21.2725) -> (-171.7675, 21.2725)
  line L1337 (-171.7675, 21.2725) -> (-171.7675, 21.9075)
  line L1338 (-171.7675, 21.9075) -> (-171.1325, 21.9075)
  line L1339 (-171.1325, 21.9075) -> (-171.1325, 21.2725)
  line L1340 (-171.1325, 18.7325) -> (-171.7675, 18.7325)
  line L1341 (-171.7675, 18.7325) -> (-171.7675, 19.3675)
  line L1342 (-171.7675, 19.3675) -> (-171.1325, 19.3675)
  line L1343 (-171.1325, 19.3675) -> (-171.1325, 18.7325)
  line L1344 (-171.1325, 16.1925) -> (-171.7675, 16.1925)
  line L1345 (-171.7675, 16.1925) -> (-171.7675, 16.8275)
  line L1346 (-171.7675, 16.8275) -> (-171.1325, 16.8275)
  line L1347 (-171.1325, 16.8275) -> (-171.1325, 16.1925)
  line L1348 (-171.1325, 13.6525) -> (-171.7675, 13.6525)
  line L1349 (-171.7675, 13.6525) -> (-171.7675, 14.2875)
  line L1350 (-171.7675, 14.2875) -> (-171.1325, 14.2875)
  line L1351 (-171.1325, 14.2875) -> (-171.1325, 13.6525)
  line L1352 (-171.1325, 11.1125) -> (-171.7675, 11.1125)
  line L1353 (-171.7675, 11.1125) -> (-171.7675, 11.7475)
  line L1354 (-171.7675, 11.7475) -> (-171.1325, 11.7475)
  line L1355 (-171.1325, 11.7475) -> (-171.1325, 11.1125)
  line L1356 (-171.1325, 8.5725) -> (-171.7675, 8.5725)
  line L1357 (-171.7675, 8.5725) -> (-171.7675, 9.2075)
  line L1358 (-171.7675, 9.2075) -> (-171.1325, 9.2075)
  line L1359 (-171.1325, 9.2075) -> (-171.1325, 8.5725)
  line L1360 (-171.1325, 6.0325) -> (-171.7675, 6.0325)
  line L1361 (-171.7675, 6.0325) -> (-171.7675, 6.6675)
  line L1362 (-171.7675, 6.6675) -> (-171.1325, 6.6675)
  line L1363 (-171.1325, 6.6675) -> (-171.1325, 6.0325)
  line L1364 (-171.1325, 3.4925) -> (-171.7675, 3.4925)
  line L1365 (-171.7675, 3.4925) -> (-171.7675, 4.1275)
  line L1366 (-171.7675, 4.1275) -> (-171.1325, 4.1275)
  line L1367 (-171.1325, 4.1275) -> (-171.1325, 3.4925)
  line L1368 (-171.1325, 0.9525) -> (-171.7675, 0.9525)
  line L1369 (-171.7675, 0.9525) -> (-171.7675, 1.5875)
  line L1370 (-171.7675, 1.5875) -> (-171.1325, 1.5875)
  line L1371 (-171.1325, 1.5875) -> (-171.1325, 0.9525)
  line L1372 (-171.1325, -1.5875) -> (-171.7675, -1.5875)
  line L1373 (-171.7675, -1.5875) -> (-171.7675, -0.9525)
  line L1374 (-171.7675, -0.9525) -> (-171.1325, -0.9525)
  line L1375 (-171.1325, -0.9525) -> (-171.1325, -1.5875)
  line L1376 (-171.1325, -4.1275) -> (-171.7675, -4.1275)
  line L1377 (-171.7675, -4.1275) -> (-171.7675, -3.4925)
  line L1378 (-171.7675, -3.4925) -> (-171.1325, -3.4925)
  line L1379 (-171.1325, -3.4925) -> (-171.1325, -4.1275)
  line L1380 (-171.1325, -6.6675) -> (-171.7675, -6.6675)
  line L1381 (-171.7675, -6.6675) -> (-171.7675, -6.0325)
  line L1382 (-171.7675, -6.0325) -> (-171.1325, -6.0325)
  line L1383 (-171.1325, -6.0325) -> (-171.1325, -6.6675)
  line L1384 (-171.1325, -9.2075) -> (-171.7675, -9.2075)
  line L1385 (-171.7675, -9.2075) -> (-171.7675, -8.5725)
  line L1386 (-171.7675, -8.5725) -> (-171.1325, -8.5725)
  line L1387 (-171.1325, -8.5725) -> (-171.1325, -9.2075)
  line L1388 (-171.1325, -11.7475) -> (-171.7675, -11.7475)
  line L1389 (-171.7675, -11.7475) -> (-171.7675, -11.1125)
  line L1390 (-171.7675, -11.1125) -> (-171.1325, -11.1125)
  line L1391 (-171.1325, -11.1125) -> (-171.1325, -11.7475)
  line L1392 (-171.1325, -14.2875) -> (-171.7675, -14.2875)
  line L1393 (-171.7675, -14.2875) -> (-171.7675, -13.6525)
  line L1394 (-171.7675, -13.6525) -> (-171.1325, -13.6525)
  line L1395 (-171.1325, -13.6525) -> (-171.1325, -14.2875)
  line L1396 (-171.1325, -16.8275) -> (-171.7675, -16.8275)
  line L1397 (-171.7675, -16.8275) -> (-171.7675, -16.1925)
  line L1398 (-171.7675, -16.1925) -> (-171.1325, -16.1925)
  line L1399 (-171.1325, -16.1925) -> (-171.1325, -16.8275)
  line L1400 (-171.1325, -19.3675) -> (-171.7675, -19.3675)
  line L1401 (-171.7675, -19.3675) -> (-171.7675, -18.7325)
  line L1402 (-171.7675, -18.7325) -> (-171.1325, -18.7325)
  line L1403 (-171.1325, -18.7325) -> (-171.1325, -19.3675)
  line L1404 (-171.1325, -21.9075) -> (-171.7675, -21.9075)
  line L1405 (-171.7675, -21.9075) -> (-171.7675, -21.2725)
  line L1406 (-171.7675, -21.2725) -> (-171.1325, -21.2725)
  line L1407 (-171.1325, -21.2725) -> (-171.1325, -21.9075)
  line L1408 (-171.1325, -24.4475) -> (-171.7675, -24.4475)
  line L1409 (-171.7675, -24.4475) -> (-171.7675, -23.8125)
  line L1410 (-171.7675, -23.8125) -> (-171.1325, -23.8125)
  line L1411 (-171.1325, -23.8125) -> (-171.1325, -24.4475)
  line L1412 (-171.1325, -26.9875) -> (-171.7675, -26.9875)
  line L1413 (-171.7675, -26.9875) -> (-171.7675, -26.3525)
  line L1414 (-171.7675, -26.3525) -> (-171.1325, -26.3525)
  line L1415 (-171.1325, -26.3525) -> (-171.1325, -26.9875)
  line L1416 (-171.1325, -29.5275) -> (-171.7675, -29.5275)
  line L1417 (-171.7675, -29.5275) -> (-171.7675, -28.8925)
  line L1418 (-171.7675, -28.8925) -> (-171.1325, -28.8925)
  line L1419 (-171.1325, -28.8925) -> (-171.1325, -29.5275)
  line L1420 (-171.1325, -32.0675) -> (-171.7675, -32.0675)
  line L1421 (-171.7675, -32.0675) -> (-171.7675, -31.4325)
  line L1422 (-171.7675, -31.4325) -> (-171.1325, -31.4325)
  line L1423 (-171.1325, -31.4325) -> (-171.1325, -32.0675)
  line L1424 (-171.1325, -34.6075) -> (-171.7675, -34.6075)
  line L1425 (-171.7675, -34.6075) -> (-171.7675, -33.9725)
  line L1426 (-171.7675, -33.9725) -> (-171.1325, -33.9725)
  line L1427 (-171.1325, -33.9725) -> (-171.1325, -34.6075)
  line L1428 (-171.1325, -37.1475) -> (-171.7675, -37.1475)
  line L1429 (-171.7675, -37.1475) -> (-171.7675, -36.5125)
  line L1430 (-171.7675, -36.5125) -> (-171.1325, -36.5125)
  line L1431 (-171.1325, -36.5125) -> (-171.1325, -37.1475)
  line L1432 (-171.1325, -39.6875) -> (-171.7675, -39.6875)
  line L1433 (-171.7675, -39.6875) -> (-171.7675, -39.0525)
  line L1434 (-171.7675, -39.0525) -> (-171.1325, -39.0525)
  line L1435 (-171.1325, -39.0525) -> (-171.1325, -39.6875)
  point P0 (0, 0)
  point P1 (170.18, 0)
  point P2 (168.91, 39.37)
  point P3 (0, -170.18)
  point P4 (0, 170.18)
  point P5 (-39.37, -171.45)
  point P6 (-36.83, -171.45)
  point P7 (-34.29, -171.45)
  point P8 (-31.75, -171.45)
  point P9 (-29.21, -171.45)
  point P10 (-26.67, -171.45)
  point P11 (-24.13, -171.45)
  point P12 (-21.59, -171.45)
  point P13 (-19.05, -171.45)
  point P14 (-16.51, -171.45)
  point P15 (-13.97, -171.45)
  point P16 (-11.43, -171.45)
  point P17 (-8.89, -171.45)
  point P18 (-6.35, -171.45)
  point P19 (-3.81, -171.45)
  point P20 (-1.27, -171.45)
  point P21 (1.27, -171.45)
  point P22 (3.81, -171.45)
  point P23 (6.35, -171.45)
  point P24 (8.89, -171.45)
  point P25 (11.43, -171.45)
  point P26 (13.97, -171.45)
  point P27 (16.51, -171.45)
  point P28 (19.05, -171.45)
  point P29 (21.59, -171.45)
  point P30 (24.13, -171.45)
  point P31 (26.67, -171.45)
  point P32 (29.21, -171.45)
  point P33 (31.75, -171.45)
  point P34 (34.29, -171.45)
  point P35 (36.83, -171.45)
  point P36 (39.37, -171.45)
  point P37 (-39.37, -168.91)
  point P38 (-36.83, -168.91)
  point P39 (-34.29, -168.91)
  point P40 (-31.75, -168.91)
  point P41 (-29.21, -168.91)
  point P42 (-26.67, -168.91)
  point P43 (-24.13, -168.91)
  point P44 (-21.59, -168.91)
  point P45 (-19.05, -168.91)
  point P46 (-16.51, -168.91)
  point P47 (-13.97, -168.91)
  point P48 (-11.43, -168.91)
  point P49 (-8.89, -168.91)
  point P50 (-6.35, -168.91)
  point P51 (-3.81, -168.91)
  point P52 (-1.27, -168.91)
  point P53 (1.27, -168.91)
  point P54 (3.81, -168.91)
  point P55 (6.35, -168.91)
  point P56 (8.89, -168.91)
  point P57 (11.43, -168.91)
  point P58 (13.97, -168.91)
  point P59 (16.51, -168.91)
  point P60 (19.05, -168.91)
  point P61 (21.59, -168.91)
  point P62 (24.13, -168.91)
  point P63 (26.67, -168.91)
  point P64 (29.21, -168.91)
  point P65 (31.75, -168.91)
  point P66 (34.29, -168.91)
  point P67 (36.83, -168.91)
  point P68 (39.37, -168.91)
  point P69 (-39.37, 168.91)
  point P70 (-36.83, 168.91)
  point P71 (-34.29, 168.91)
  point P72 (-31.75, 168.91)
  point P73 (-29.21, 168.91)
  point P74 (-26.67, 168.91)
  point P75 (-24.13, 168.91)
  point P76 (-21.59, 168.91)
  point P77 (-19.05, 168.91)
  point P78 (-16.51, 168.91)
  point P79 (-13.97, 168.91)
  point P80 (-11.43, 168.91)
  point P81 (-8.89, 168.91)
  point P82 (-6.35, 168.91)
  point P83 (-3.81, 168.91)
  point P84 (-1.27, 168.91)
  point P85 (1.27, 168.91)
  point P86 (3.81, 168.91)
  point P87 (6.35, 168.91)
  point P88 (8.89, 168.91)
  point P89 (11.43, 168.91)
  point P90 (13.97, 168.91)
  point P91 (16.51, 168.91)
  point P92 (19.05, 168.91)
  point P93 (21.59, 168.91)
  point P94 (24.13, 168.91)
  point P95 (26.67, 168.91)
  point P96 (29.21, 168.91)
  point P97 (31.75, 168.91)
  point P98 (34.29, 168.91)
  point P99 (36.83, 168.91)
  point P100 (39.37, 168.91)
  point P101 (-39.37, 171.45)
  point P102 (-36.83, 171.45)
  point P103 (-34.29, 171.45)
  point P104 (-31.75, 171.45)
  point P105 (-29.21, 171.45)
  point P106 (-26.67, 171.45)
  point P107 (-24.13, 171.45)
  point P108 (-21.59, 171.45)
  point P109 (-19.05, 171.45)
  point P110 (-16.51, 171.45)
  point P111 (-13.97, 171.45)
  point P112 (-11.43, 171.45)
  point P113 (-8.89, 171.45)
  point P114 (-6.35, 171.45)
  point P115 (-3.81, 171.45)
  point P116 (-1.27, 171.45)
  point P117 (1.27, 171.45)
  point P118 (3.81, 171.45)
  point P119 (6.35, 171.45)
  point P120 (8.89, 171.45)
  point P121 (11.43, 171.45)
  point P122 (13.97, 171.45)
  point P123 (16.51, 171.45)
  point P124 (19.05, 171.45)
  point P125 (21.59, 171.45)
  point P126 (24.13, 171.45)
  point P127 (26.67, 171.45)
  point P128 (29.21, 171.45)
  point P129 (31.75, 171.45)
  point P130 (34.29, 171.45)
  point P131 (36.83, 171.45)
  point P132 (39.37, 171.45)
  point P133 (168.91, 36.83)
  point P134 (168.91, 34.29)
  point P135 (168.91, 31.75)
  point P136 (168.91, 29.21)
  point P137 (168.91, 26.67)
  point P138 (168.91, 24.13)
  point P139 (168.91, 21.59)
  point P140 (168.91, 19.05)
  point P141 (168.91, 16.51)
  point P142 (168.91, 13.97)
  point P143 (168.91, 11.43)
  point P144 (168.91, 8.89)
  point P145 (168.91, 6.35)
  point P146 (168.91, 3.81)
  point P147 (168.91, 1.27)
  point P148 (168.91, -1.27)
  point P149 (168.91, -3.81)
  point P150 (168.91, -6.35)
  point P151 (168.91, -8.89)
  point P152 (168.91, -11.43)
  point P153 (168.91, -13.97)
  point P154 (168.91, -16.51)
  point P155 (168.91, -19.05)
  point P156 (168.91, -21.59)
  point P157 (168.91, -24.13)
  point P158 (168.91, -26.67)
  point P159 (168.91, -29.21)
  point P160 (168.91, -31.75)
  point P161 (168.91, -34.29)
  point P162 (168.91, -36.83)
  point P163 (168.91, -39.37)
  point P164 (171.45, 39.37)
  point P165 (171.45, 36.83)
  point P166 (171.45, 34.29)
  point P167 (171.45, 31.75)
  point P168 (171.45, 29.21)
  point P169 (171.45, 26.67)
  point P170 (171.45, 24.13)
  point P171 (171.45, 21.59)
  point P172 (171.45, 19.05)
  point P173 (171.45, 16.51)
  point P174 (171.45, 13.97)
  point P175 (171.45, 11.43)
  point P176 (171.45, 8.89)
  point P177 (171.45, 6.35)
  point P178 (171.45, 3.81)
  point P179 (171.45, 1.27)
  point P180 (171.45, -1.27)
  point P181 (171.45, -3.81)
  point P182 (171.45, -6.35)
  point P183 (171.45, -8.89)
  point P184 (171.45, -11.43)
  point P185 (171.45, -13.97)
  point P186 (171.45, -16.51)
  point P187 (171.45, -19.05)
  point P188 (171.45, -21.59)
  point P189 (171.45, -24.13)
  point P190 (171.45, -26.67)
  point P191 (171.45, -29.21)
  point P192 (171.45, -31.75)
  point P193 (171.45, -34.29)
  point P194 (171.45, -36.83)
  point P195 (171.45, -39.37)
  dimension "d52" = 5.08
  dimension "d109" = 5.08
  dimension "d110" = 81.28
  dimension "d112" = 5.08
  dimension "d113" = 0
  dimension "d119" = 0
  dimension "d120" = 5.08
  dimension "d122" = 0.635
  dimension "d130" = 2.54
  dimension "d133" = 2.54
  dimension "d139" = 1.27
  dimension "d140" = 1.27
  dimension "d142" = 1.27
  dimension "d143" = 1.27
  dimension "d144" = 1.27
  dimension "d145" = 1.27
  dimension "d148" = 2.54
  dimension "d151" = 2.54
  dimension "d156" = 2.54
  dimension "d159" = 2.54
  dimension "d182" = 2.54
  dimension "d185" = 2.54
  constraints: 2860 end point, 390 midpoint, 12 parallel, 10 horizontal, 9 equal length, 8 symmetric about line, 6 perpendicular, 4 vertical, 1 point on line, 2583 other
  measures "d52" distance between parallel lines of L4 L7
  measures "d109" distance of L19.end L17.start
  measures "d110" distance of L17.start L17.end
  measures "d112" distance between parallel lines of L23 L19
  measures "d113" distance from line of L16 point (0, -170.18)
  measures "d119" distance from line of L16 point (0, 170.18)
  measures "d120" distance between parallel lines of L8 L24
  measures "d122" distance of L31.end L32.end
  measures "d130" distance of L30.start L36.start
  measures "d133" distance of L30.start L222.start
  measures "d139" distance from line of L18 point (-39.37, -171.45)
  measures "d140" distance from line of L19 point (-39.37, -171.45)
  measures "d142" distance from line of L2 point (168.91, 39.37)
  measures "d143" distance from line of L3 point (168.91, 39.37)
  measures "d144" distance from line of L25 point (-39.37, 168.91)
  measures "d145" distance from line of L26 point (-39.37, 168.91)
  measures "d148" distance of L415.end L420.start
  measures "d151" distance of L415.end L606.start
  measures "d156" distance of L10.start L798.start
  measures "d159" distance of L10.start L984.start
  measures "d182" distance of L1182.start L1184.start
  measures "d185" distance of L1182.start L1308.start